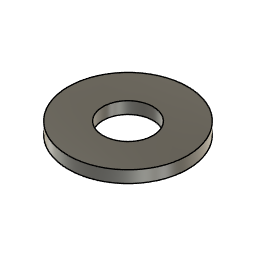
Spacer v4 (Autodesk Fusion 360 design; units mm, degrees)
Autodesk Fusion 360 part; units mm, degrees
sketch "Esboço3" plane through (0, 0, 0) normal (0, 0, 1) x (1, 0, 0)
  circle A0 centre (0, 0) radius 5
  dimension "d7" = 10
  constraint coincident A0.centre origin
  measures "d7" diameter of A0
extrude "Extrusão3" add sketch "Esboço3" along normal blind 1
sketch "Esboço4" plane through (0, 0, 1) normal (0, 0, 1) x (-1, 0, 0)
  circle A0 centre (0, 0) radius 5
  circle A1 centre (0, 0) radius 2.1
  dimension "d10" = 4.2
  constraint coincident A0.centre A1.centre
  measures "d10" diameter of A1
extrude "Extrusão4" cut sketch "Esboço4" against normal blind 5 contours A1
